# Autodesk Inventor part: A3.3
Saved by Autodesk Inventor 2023 (Build 270158000, 158)
## iProperties
Created: 2023-04-05
Part Number: A3.3
Material: Generic
Document SubType Name: Modeling
Standard: ME4Z03
Designer: Steven
Manufacturer: McMaster University
Language: en-US
Size Designation: (Unnamed 1)
Categories: <MemberInstance><Categories><Category DisplayName="Structural Shapes" InternalName="089c4875-fa83-4c05-b084-43b9cc11f5ed" Mnemonic="GRDR"><CategoryParameter DisplayName="Mass per Length Unit" InternalName="0bb95a10-148f-4027-a459-38d7b056702a" Mnemonic="shpmass"/><CategoryParameter DisplayName="Section Area" InternalName="1ff91680-64b0-4202-b9a3-7fd3f94bba3b" Mnemonic="secarea"/><CategoryParameter DisplayName="Radius of Gyration (x)" InternalName="25778675-03e9-40c1-b6a8-4a9ed693320d" Mnemonic="gyrradx"/><CategoryParameter DisplayName="Torsional Rigidity Modulus" InternalName="26c1ec35-5026-4c63-ad0a-751cf684a536" Mnemonic="torrigmod"/><CategoryParameter DisplayName="Distance of the Center of Gravity X-X" InternalName="26c9bdb8-9c79-4b4f-a92e-8e197583c9c4" Mnemonic="grcendistX"/><CategoryParameter DisplayName="Legacy Member ID" InternalName="340afe4f-75d7-48d3-ab7d-943f3c3da468" Mnemonic="LegacyMemberID"/><CategoryParameter DisplayName="Base Length" InternalName="42e34263-8f20-4d0e-ad48-bf1385b87c24" Mnemonic="shplen"/><CategoryParameter DisplayName="Moment of Inertia (y)" InternalName="4b9f58ea-bced-460e-81ea-3d29ca5a49e3" Mnemonic="inermomy"/><CategoryParameter DisplayName="Moment of Inertia (x)" InternalName="4cd780bc-73d7-43ac-917a-579e5cbd684d" Mnemonic="inermomx"/><CategoryParameter DisplayName="Custom Base Point" InternalName="4f1d1b73-316d-484b-a3df-9cbabb16eb77" Mnemonic="shpBasePoint"/><CategoryParameter DisplayName="Shape Height" InternalName="50274e7d-5ac0-4796-92cb-c59e54983c67" Mnemonic="shpheig"/><CategoryParameter DisplayName="Section Module (y)" InternalName="59eaa5e9-d227-48dc-b6c1-6920f96e0f95" Mnemonic="secmody"/><CategoryParameter DisplayName="Section Designation" InternalName="5a64d034-428d-49c8-ba32-7619764de20f" Mnemonic="shpdes"/><CategoryParameter DisplayName="Section Module (x)" InternalName="72cfad18-cf51-4ed4-aaa7-c6b224f8419f" Mnemonic="secmodx"/><CategoryParameter DisplayName="Torsional Section Modulus" InternalName="7c55a8dc-8844-49f9-a867-cc677b30ec9a" Mnemonic="torsecmod"/><CategoryParameter DisplayName="Shape Width" InternalName="7c717d54-a18f-4666-b4d4-573cce22c62c" Mnemonic="shpwdth"/><CategoryParameter DisplayName="Second Shape Thickness" InternalName="9251a8e1-85fd-4e47-af99-afdb762317d9" Mnemonic="shpthick2"/><CategoryParameter DisplayName="FG Authored" InternalName="9c666724-f362-4ea7-ac62-f6a007de5c69" Mnemonic="shpFGAuto"/><CategoryParameter DisplayName="Distance of the Center of Gravity Y-Y" InternalName="bcc4fb17-7af4-436a-8f8c-d0aa3b0248c5" Mnemonic="grcendistY"/><CategoryParameter DisplayName="Radius of Gyration (y)" InternalName="bfa18ebe-1636-4dbe-8d42-b263e0b73184" Mnemonic="gyrrady"/><CategoryParameter DisplayName="Shape Thickness" InternalName="d109cf76-8eb4-42fc-9800-4409734adc67" Mnemonic="shpthick"/><CategoryParameter DisplayName="Coefficient of Shear Displacement" InternalName="de4c90c6-aaa8-468f-a335-6737b311b5d3" Mnemonic="shdispc"/><Category DisplayName="Other" InternalName="f02205ff-2390-476f-921c-0b3185f88e84" Mnemonic="OTHSHP"><CategoryParameter DisplayName="Moment of Inertia (y)" InternalName="044c654e-f649-48ac-84cc-650a29ae31ca" Mnemonic="inermomy"/><CategoryParameter DisplayName="Shape Thickness" InternalName="12b1a788-9233-48fd-a933-2df8ff42b15f" Mnemonic="shpthick"/><CategoryParameter DisplayName="Mass per Length Unit" InternalName="2fd289d6-9394-4d2d-97e6-6659d7d4551d" Mnemonic="shpmass"/><CategoryParameter DisplayName="Radius of Gyration (y)" InternalName="743e1dfe-1bba-408b-b985-cf752b207386" Mnemonic="gyrrady"/><CategoryParameter DisplayName="Section Module (y)" InternalName="88b8bff9-a616-4028-93d5-ed4f79680d13" Mnemonic="secmody"/><CategoryParameter DisplayName="Section Area" InternalName="c46ecdf8-b6eb-4db9-8b25-30258930c1e3" Mnemonic="secarea"/><CategoryParameter DisplayName="Section Module (x)" InternalName="cac70804-9d39-43bb-be17-56ea1f39a6c2" Mnemonic="secmodx"/><CategoryParameter DisplayName="Moment of Inertia (x)" InternalName="ec6737bc-264f-43ed-b0bd-f6d410c2718d" Mnemonic="inermomx"/><CategoryParameter DisplayName="Radius of Gyration (x)" InternalName="ee72c61e-565e-4fd6-b448-66e1e1abcb7e" Mnemonic="gyrradx"/></Category></Category><Category DisplayName="DataType" InternalName="23b78d0f-2648-40c6-8793-ca6db495c9e8" Mnemonic="DATATYPE"><CategoryParameter DisplayName="DisplayName" InternalName="05415f3d-3907-474b-a020-eb9d644f4cf3" Mnemonic="DISPLAYNAME"/><CategoryParameter DisplayName="Standard" InternalName="0c0a119c-1e12-4c84-803f-101930972f5e" Mnemonic="STANDARD"/><CategoryParameter DisplayName="Description" InternalName="13903e3d-64b1-4950-80da-f627842ea37f" Mnemonic="DESCRIPTION"/><CategoryParameter DisplayName="Designation" InternalName="2675968c-4ce5-49e0-a4f5-552d29089031" Mnemonic="DESIGNATION"/><CategoryParameter DisplayName="Default Row" InternalName="2af9ec52-faaa-4026-b378-f9fa4afca842" Mnemonic="DEFAULTROW"/><CategoryParameter DisplayName="Folder Name" InternalName="3f06958e-8713-4116-9be7-ed6184ecc97b" Mnemonic="FOLDERNAME"/><CategoryParameter DisplayName="Revision Guid" InternalName="45a75005-10b1-4dfc-8d6d-dfe629f0b93c" Mnemonic="REVISIONGUID"/><CategoryParameter DisplayName="FileName" InternalName="8b46a4cc-9585-4fed-90c3-899f57e09a73" Mnemonic="FILENAME"/><CategoryParameter DisplayName="StdsOrg" InternalName="8f5914e1-4693-403f-8ab5-d37768198c9d" Mnemonic="STDSORG"/><CategoryParameter DisplayName="Family Version" InternalName="914462f6-6e19-4b14-ba84-155b9680b1d0" Mnemonic="FAMILYREVISION"/><CategoryParameter DisplayName="Standard Revision" InternalName="91d5a463-65c2-4fde-b823-3b7fea5e8e17" Mnemonic="STANDARDREVISION"/><CategoryParameter DisplayName="Member Revision" InternalName="a65d44b9-392f-4f4f-857b-e4b3d54996fe" Mnemonic="MEMBERREVISION"/><CategoryParameter DisplayName="ClipFormat" InternalName="bc51e27b-3422-4e78-93ef-cec197ddf230" Mnemonic="CLIPFORMAT"/><CategoryParameter DisplayName="Manufacturer" InternalName="cd6c7a72-a28a-4e50-99a9-2c7f4e13e5ad" Mnemonic="MANUFACTURER"/><CategoryParameter DisplayName="InternalName" InternalName="cf1d0246-76d9-4b4a-8305-fa0409afb5c1" Mnemonic="INTERNALNAME"/><CategoryParameter DisplayName="IsMetric" InternalName="e2385c5b-1ea4-4823-96a8-8de651266ec3" Mnemonic="ISMETRIC"/><Category DisplayName="Part" InternalName="c0e0b642-3bcb-4cc8-9e80-f96d35c4afa4" Mnemonic="PART"><CategoryParameter DisplayName="Part Number" InternalName="016b6077-bfbe-49bd-92c9-d8d59c39c941" Mnemonic="PARTNUMBER"/><CategoryParameter DisplayName="Stock Number" InternalName="4dba7c1c-e26c-444e-836c-b08b433409a8" Mnemonic="STOCKNUMBER"/><CategoryParameter DisplayName="Material Key" InternalName="5c9a8adb-dd2b-4535-b97f-0a94a95fe41f" Mnemonic="MATERIALKEY"/><CategoryParameter DisplayName="Material" InternalName="818a152a-d3c3-49ca-80ee-df7d91421b8e" Mnemonic="MATERIAL"/></Category></Category></Categories><FamilyTemplate Id="A3.3"><FamilyTemplateParameters><FamilyTemplateParameter ObjectType="kModelParameterObject" ValueType="xs:double" Id="12" ObjectReferenceKey="Length"/><FamilyTemplateParameter ObjectType="kPartComponentDefinitionObject" ValueType="xs:string" Id="23" SubObjectId="Material"/><FamilyTemplateParameter ObjectType="kPropertyObject" ValueType="xs:string" Id="26" ObjectReferenceKey="{32853F0F-3444-11d1-9E93-0060B03C1CA6}" SubObjectId="5"/><FamilyTemplateParameter ObjectType="kPropertyObject" ValueType="xs:string" Id="27" ObjectReferenceKey="{32853F0F-3444-11d1-9E93-0060B03C1CA6}" SubObjectId="52"/></FamilyTemplateParameters></FamilyTemplate><CategoryParameterMap><ParamToTemplateMap><ParamToTemplate CategoryParameter="//CategoryParameter[@InternalName='cf1d0246-76d9-4b4a-8305-fa0409afb5c1']" ConstantValue="c2515e16-9b14-40ac-b273-dfd0c39fec72"/><ParamToTemplate CategoryParameter="//CategoryParameter[@InternalName='45a75005-10b1-4dfc-8d6d-dfe629f0b93c']" ConstantValue="d7c3d587-e6b2-49f4-a210-89fb3e91c4c4"/><ParamToTemplate CategoryParameter="//CategoryParameter[@InternalName='3f06958e-8713-4116-9be7-ed6184ecc97b']" ConstantValue="A3.3"/><ParamToTemplate CategoryParameter="//CategoryParameter[@InternalName='8f5914e1-4693-403f-8ab5-d37768198c9d']" TemplateParameter="17"/><ParamToTemplate CategoryParameter="//CategoryParameter[@InternalName='0c0a119c-1e12-4c84-803f-101930972f5e']" ConstantValue="ME4Z03"/><ParamToTemplate CategoryParameter="//CategoryParameter[@InternalName='91d5a463-65c2-4fde-b823-3b7fea5e8e17']" TemplateParameter="19"/><ParamToTemplate CategoryParameter="//CategoryParameter[@InternalName='cd6c7a72-a28a-4e50-99a9-2c7f4e13e5ad']" ConstantValue="McMaster University"/><ParamToTemplate CategoryParameter="//CategoryParameter[@InternalName='13903e3d-64b1-4950-80da-f627842ea37f']" TemplateParameter="22"/><ParamToTemplate CategoryParameter="//CategoryParameter[@InternalName='05415f3d-3907-474b-a020-eb9d644f4cf3']" ConstantValue="A3.3"/><ParamToTemplate CategoryParameter="//CategoryParameter[@InternalName='914462f6-6e19-4b14-ba84-155b9680b1d0']" ConstantValue="11"/><ParamToTemplate CategoryParameter="//CategoryParameter[@InternalName='bc51e27b-3422-4e78-93ef-cec197ddf230']" ConstantValue="CF_INVENTOR.STDPARTS"/><ParamToTemplate CategoryParameter="//CategoryParameter[@InternalName='e2385c5b-1ea4-4823-96a8-8de651266ec3']" ConstantValue="true"/><ParamToTemplate CategoryParameter="//CategoryParameter[@InternalName='2af9ec52-faaa-4026-b378-f9fa4afca842']" ConstantValue="1"/><ParamToTemplate CategoryParameter="//CategoryParameter[@InternalName='9c666724-f362-4ea7-ac62-f6a007de5c69']" ConstantValue="1"/><ParamToTemplate CategoryParameter="//CategoryParameter[@InternalName='8b46a4cc-9585-4fed-90c3-899f57e09a73']" ConstantValue="100"/><ParamToTemplate CategoryParameter="//CategoryParameter[@InternalName='a65d44b9-392f-4f4f-857b-e4b3d54996fe']" ConstantValue="9465c23e-afda-41ef-8d3f-85a5f6d5f641"/><ParamToTemplate CategoryParameter="//CategoryParameter[@InternalName='a65d44b9-392f-4f4f-857b-e4b3d54996fe']" ConstantValue="9465c23e-afda-41ef-8d3f-85a5f6d5f641"/><ParamToTemplate CategoryParameter="//CategoryParameter[@InternalName='2675968c-4ce5-49e0-a4f5-552d29089031']" TemplateParameter="27"/><ParamToTemplate CategoryParameter="//CategoryParameter[@InternalName='42e34263-8f20-4d0e-ad48-bf1385b87c24']" TemplateParameter="12"/><ParamToTemplate CategoryParameter="//CategoryParameter[@InternalName='818a152a-d3c3-49ca-80ee-df7d91421b8e']" TemplateParameter="23"/><ParamToTemplate CategoryParameter="//CategoryParameter[@InternalName='016b6077-bfbe-49bd-92c9-d8d59c39c941']" TemplateParameter="26"/></ParamToTemplateMap></CategoryParameterMap></MemberInstance>
Density: 1 g/cm^3
Appearance: Default
IsCustomPart: 1
G_L: 284.800 mm
G_W: 20.000 mm
G_H: 20.000 mm
+DF7D714F-C0FD-47DF-899F-53EAE2607CEB+CUTDETAIL1: Cut Angle 90.00 deg
+4205FE6B-57FF-4639-AF32-875A4B7A86CD+CUTDETAIL2: Cut Angle 90.00 deg
_CCFamilyDisplayName: A3.3
_FrameMemberDoc: Frame Member File
_Version: 25.0.0
_GetPNFromCC: 1
Author: Steven
Autodesk Inventor part; units mm, degrees
ref_plane "Start Plane" through (0, 10, 0) normal (0, 1, 0) x (-1, 0, 0)
ref_plane "End Plane" through (0, 294.8, 0) normal (0, 1, 0) x (-1, 0, 0)
sketch "Sketch" plane through (0, 0, 0) normal (0, 1, 0) x (-1, 0, 0)
  line L0 (-1.7574, 4) -> (1.7574, 4)
  line L1 (4, 1.7574) -> (4, -1.7574)
  line L2 (1.7574, -4) -> (-1.7574, -4)
  line L3 (-4, -1.7574) -> (-4, 1.7574)
  line L4 (4.5858, -3.1716) -> (7.1464, -5.7322)
  line L5 (3.1716, -4.5858) -> (5.7322, -7.1464)
  line L6 (5.3787, -8) -> (3.5, -8)
  line L7 (3, -8.5) -> (3, -9.5)
  line L8 (3.5, -10) -> (9, -10)
  line L9 (10, -9) -> (10, -3.5)
  line L10 (9.5, -3) -> (8.5, -3)
  line L11 (8, -3.5) -> (8, -5.3787)
  line L12 (4, 0) -> (-4, 0) construction
  line L13 (0, -4) -> (0, 4) construction
  arc A0 (4, -1.7574) -> (4.5858, -3.1716) centre (6, -1.7574) ccw
  arc A1 (3.1716, -4.5858) -> (1.7574, -4) centre (1.7574, -6) ccw
  arc A2 (3.5, -8) -> (3, -8.5) centre (3.5, -8.5) ccw
  arc A3 (3, -9.5) -> (3.5, -10) centre (3.5, -9.5) ccw
  arc A4 (10, -3.5) -> (9.5, -3) centre (9.5, -3.5) ccw
  arc A5 (8.5, -3) -> (8, -3.5) centre (8.5, -3.5) ccw
  arc A6 (7.1464, -5.7322) -> (8, -5.3787) centre (7.5, -5.3787) ccw
  arc A7 (5.3787, -8) -> (5.7322, -7.1464) centre (5.3787, -7.5) ccw
  arc A8 (9, -10) -> (10, -9) centre (9, -9) ccw
  line L14 (-4.5858, -3.1716) -> (-7.1464, -5.7322)
  line L15 (-3.1716, -4.5858) -> (-5.7322, -7.1464)
  line L16 (-5.3787, -8) -> (-3.5, -8)
  line L17 (-3, -8.5) -> (-3, -9.5)
  line L18 (-3.5, -10) -> (-9, -10)
  line L19 (-10, -9) -> (-10, -3.5)
  line L20 (-9.5, -3) -> (-8.5, -3)
  line L21 (-8, -3.5) -> (-8, -5.3787)
  arc A9 (-4.5858, -3.1716) -> (-4, -1.7574) centre (-6, -1.7574) ccw
  arc A10 (-1.7574, -4) -> (-3.1716, -4.5858) centre (-1.7574, -6) ccw
  arc A11 (-3, -8.5) -> (-3.5, -8) centre (-3.5, -8.5) ccw
  arc A12 (-3.5, -10) -> (-3, -9.5) centre (-3.5, -9.5) ccw
  arc A13 (-9.5, -3) -> (-10, -3.5) centre (-9.5, -3.5) ccw
  arc A14 (-8, -3.5) -> (-8.5, -3) centre (-8.5, -3.5) ccw
  arc A15 (-8, -5.3787) -> (-7.1464, -5.7322) centre (-7.5, -5.3787) ccw
  arc A16 (-5.7322, -7.1464) -> (-5.3787, -8) centre (-5.3787, -7.5) ccw
  arc A17 (-10, -9) -> (-9, -10) centre (-9, -9) ccw
  line L22 (4.5858, 3.1716) -> (7.1464, 5.7322)
  line L23 (3.1716, 4.5858) -> (5.7322, 7.1464)
  line L24 (5.3787, 8) -> (3.5, 8)
  line L25 (3, 8.5) -> (3, 9.5)
  line L26 (3.5, 10) -> (9, 10)
  line L27 (10, 9) -> (10, 3.5)
  line L28 (9.5, 3) -> (8.5, 3)
  line L29 (8, 3.5) -> (8, 5.3787)
  arc A18 (4.5858, 3.1716) -> (4, 1.7574) centre (6, 1.7574) ccw
  arc A19 (1.7574, 4) -> (3.1716, 4.5858) centre (1.7574, 6) ccw
  arc A20 (3, 8.5) -> (3.5, 8) centre (3.5, 8.5) ccw
  arc A21 (3.5, 10) -> (3, 9.5) centre (3.5, 9.5) ccw
  arc A22 (9.5, 3) -> (10, 3.5) centre (9.5, 3.5) ccw
  arc A23 (8, 3.5) -> (8.5, 3) centre (8.5, 3.5) ccw
  arc A24 (8, 5.3787) -> (7.1464, 5.7322) centre (7.5, 5.3787) ccw
  arc A25 (5.7322, 7.1464) -> (5.3787, 8) centre (5.3787, 7.5) ccw
  arc A26 (10, 9) -> (9, 10) centre (9, 9) ccw
  line L30 (-10, 9) -> (-10, 3.5)
  arc A27 (-9, 10) -> (-10, 9) centre (-9, 9) ccw
  arc A28 (-10, 3.5) -> (-9.5, 3) centre (-9.5, 3.5) ccw
  line L31 (-9.5, 3) -> (-8.5, 3)
  arc A29 (-8.5, 3) -> (-8, 3.5) centre (-8.5, 3.5) ccw
  line L32 (-8, 3.5) -> (-8, 5.3787)
  arc A30 (-7.1464, 5.7322) -> (-8, 5.3787) centre (-7.5, 5.3787) ccw
  line L33 (-4.5858, 3.1716) -> (-7.1464, 5.7322)
  line L34 (-3.1716, 4.5858) -> (-5.7322, 7.1464)
  arc A31 (-3.1716, 4.5858) -> (-1.7574, 4) centre (-1.7574, 6) ccw
  arc A32 (-4, 1.7574) -> (-4.5858, 3.1716) centre (-6, 1.7574) ccw
  arc A33 (-5.3787, 8) -> (-5.7322, 7.1464) centre (-5.3787, 7.5) ccw
  line L35 (-5.3787, 8) -> (-3.5, 8)
  arc A34 (-3.5, 8) -> (-3, 8.5) centre (-3.5, 8.5) ccw
  line L36 (-3, 8.5) -> (-3, 9.5)
  arc A35 (-3, 9.5) -> (-3.5, 10) centre (-3.5, 9.5) ccw
  line L37 (-3.5, 10) -> (-9, 10)
  circle A36 centre (0, 0) radius 2.5
  point P0 (3, -8)
  point P1 (3, -10)
  point P2 (10, -10)
  dimension "d3" = 2
  dimension "d4" = 2
  dimension "d5" = 7
  dimension "d6" = 2
  dimension "d7" = 0.5
  dimension "d8" = 1
  dimension "d9" = 20
  dimension "d10" = 20
  dimension "d11" = 8
  dimension "d13" = 5
  dimension "d14" = 8
  constraints: 81 symmetric about line, 76 end point, 72 point on circle, 37 centre point, 18 tangent, 6 equal radius, 6 midpoint, 6 point on line, 5 perpendicular, 4 equal length, 3 horizontal, 3 parallel, 2 coincident, 2 vertical, 27 other
  measures "d3" distance between parallel lines of L5 L4
  measures "d4" distance of point (3, -8) point (3, -10)
  measures "d5" distance of point (10, -10) point (3, -10)
  measures "d6" radius of A0
  measures "d7" radius of A2
  measures "d8" radius of A8
  measures "d9" distance between parallel lines of L30 L27
  measures "d10" distance between parallel lines of L8 L26
  measures "d11" distance between parallel lines of L3 L1
  measures "d13" diameter of A36
  measures "d14" distance between parallel lines of L0 L2
extrude "Body" add sketch "Sketch" along normal up to surface (284.8 mm away) from surface at 10
sketch "Sketch4" plane through (0, 0, 0) normal (0, 1, 0) x (-1, 0, 0)
  line L0 (0, 0) -> (10, 0)
ref_plane "Work Plane4" through (0, 0, 0) normal (0, 0, -1) x (-1, 0, 0)
sketch "Sketch5" plane through (0, 0, 0) normal (0, 0, -1) x (-1, 0, 0)
  line L0 (-2, 10) -> (12, 10)
  line L1 (-2, 294.8) -> (12, 294.8)
  dimension "d22" = 284.8
  measures "d22" distance between parallel lines of L0 L1
ref_plane "Work Plane5" through (0, 294.8, 3.5) normal (0, 1, 0) x (1, 0, 0)
split "Split1" plane through (0, 294.8, 3.5) removes the side toward (0, 1, 0)
ref_plane "Work Plane6" through (-279.4, 10, 3.5) normal (0, -1, 0) x (1, 0, 0)
split "Split2" plane through (-279.4, 10, 3.5) removes the side toward (0, -1, 0)
equation "\"d18\" = Length + G_OFFSET_END"
equation "\"G_L\" = d22"
equation "\"Length\" = 304.8"
equation "\"G_OFFSET_END\" = -10"
body "Solid1"
